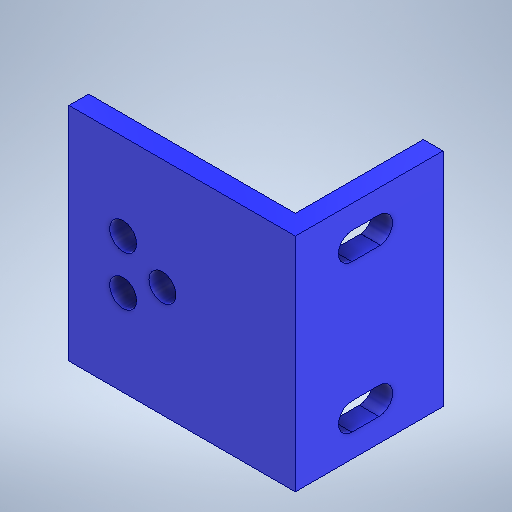
# Autodesk Inventor part: Montagewinkel für Spannelement
Saved by Autodesk Inventor 2025.1 (Build 291241020, 241B)
## iProperties
Created: 2026-05-13
Part Number: Montagewinkel für Spannelement
Material: Generisch
Document SubType Name: Modeling
Designer: pparr
Density: 1 g/cm^3
Appearance: Blau - Wandfarbe - glänzend
Author: pparr
Autodesk Inventor part; units mm, degrees
ref_plane "YZ Plane" through (0, 0, 0) normal (1, 0, 0) x (0, 1, 0)
ref_plane "XZ Plane" through (0, 0, 0) normal (0, 1, 0) x (-1, 0, 0)
ref_plane "XY Plane" through (0, 0, 0) normal (0, 0, 1) x (1, 0, 0)
sketch "Skizze1" plane through (0, 0, 0) normal (1, 0, 0) x (0, 1, 0)
  line L0 (15, 22.5) -> (-15, 22.5)
  line L1 (-15, 22.5) -> (-15, -22.5)
  line L2 (-15, -22.5) -> (15, -22.5)
  line L3 (15, -22.5) -> (15, 22.5)
  line L4 (15, 22.5) -> (-15, -22.5) construction
  line L5 (-15, 22.5) -> (15, -22.5) construction
  point P0 (0, 0)
  dimension "d0" = 30
  dimension "d1" = 45
  constraints: 12 end point, 2 midpoint, 2 parallel, 1 horizontal, 1 perpendicular
  measures "d0" distance of L2.end L1.end
  measures "d1" distance of L1.end L0.end
extrude "Extrusion1" add sketch "Skizze1" along normal blind 4
sketch "Skizze2" plane through (0, 0, 0) normal (-1, 0, 0) x (0, 0, 1)
  line L0 (-22.5, -15) -> (-22.5, 15) projected
  line L1 (-22.5, -11) -> (22.5, -11)
  line L2 (22.5, -11) -> (22.5, -15)
  line L3 (22.5, -15) -> (-22.5, -15)
  line L4 (-22.5, -15) -> (-22.5, -11)
  line L5 (22.5, -15) -> (-22.5, -15) projected
  point P0 (0, 0)
  dimension "d4" = 4
  dimension "d5" = 0
  constraints: 8 end point, 2 parallel, 1 horizontal, 1 perpendicular, 1 point on line
  measures "d4" distance of L1.end L2.end
  measures "d5" distance between parallel lines of L5 L3
extrude "Extrusion2" add sketch "Skizze2" along normal blind 42
sketch "Skizze3" plane through (4, -15, -22.5) normal (0, -1, 0) x (1, 0, 0)
  line L0 (0, 22.5) -> (-45.8958, 22.5)
  line L1 (0, 45) -> (0, 0) projected
  line L2 (-46, 0) -> (-46, 45) projected
  point P0 (-4, 22.5)
  point P1 (-27, 22.5)
  point P2 (-35, 17.5)
  point P3 (-35, 27.5)
  point P4 (-46, 22.5)
  dimension "d15" = 27
  dimension "d17" = 10
  dimension "d18" = 35
  dimension "d19" = 0
  dimension "d21" = 5
  constraints: 2 end point, 2 midpoint, 1 horizontal, 1 point on line
  measures "d15" distance from line of L1 point (-27, 22.5)
  measures "d17" distance of point (-35, 27.5) point (-35, 17.5)
  measures "d18" horizontal distance of point (-35, 17.5) L1.end
  measures "d19" horizontal distance of point (-35, 17.5) point (-35, 27.5)
  measures "d21" vertical distance of point (-35, 17.5) point (-46, 22.5)
hole "Bohrung1" at (-23, -15, 0) at (-31, -15, -5) at (-31, -15, 5) direction (0, 1, 0) diameter 5.5 depth 11.8 tip angle 118
sketch "Skizze5" plane through (0, 0, 0) normal (-1, 0, 0) x (0, 0, 1)
  line L0 (-22.5, -15) -> (22.5, -15) projected
  point P0 (0, 0)
  point P1 (15, -3.5)
  point P2 (-15, -3.5)
  point P3 (15, 2)
  point P4 (-15, 2)
  dimension "d29" = 30
  dimension "d30" = 15
  dimension "d31" = 11.5
  dimension "d32" = 11.5
  dimension "d33" = 15
  dimension "d34" = 30
  dimension "d35" = 5.5
  dimension "d36" = 5.5
  measures "d29" distance of point (-15, -3.5) point (15, -3.5)
  measures "d30" horizontal distance of point (15, -3.5) point (0, 0)
  measures "d31" distance from line of point (15, -3.5) L0
  measures "d32" distance from line of L0 point (-15, -3.5)
  measures "d33" horizontal distance of point (0, 0) point (15, 2)
  measures "d34" distance of point (-15, 2) point (15, 2)
  measures "d35" distance of point (15, 2) point (15, -3.5)
  measures "d36" distance of point (-15, -3.5) point (-15, 2)
hole "Bohrung2" at (0, -3.5, 15) at (0, -3.5, -15) at (0, 2, 15) at (0, 2, -15) direction (1, 0, 0) diameter 5.5 depth 11.8 tip angle 118
sketch "Skizze6" plane through (0, 0, 0) normal (-1, 0, 0) x (0, 0, 1)
  circle A0 centre (15, -3.5) radius 2.75 projected
  line L0 (17.75, -3.5) -> (17.75, 2.2896)
  line L1 (12.25, -3.5) -> (12.25, 2.2896)
  circle A1 centre (-15, -3.5) radius 2.75 projected
  line L2 (-12.25, -3.5) -> (-12.25, 2.2896)
  line L3 (-17.75, -3.5) -> (-17.75, 2)
  circle A2 centre (-15, 2) radius 2.75 projected
  line L4 (17.75, -3.5) -> (12.25, -3.5)
  line L5 (17.75, 2.2896) -> (12.25, 2.2896)
  line L6 (-12.25, -3.5) -> (-17.75, -3.5)
  line L7 (-12.25, 2.2896) -> (-17.7347, 2.2896)
  circle A3 centre (-15, 2) radius 2.75 projected
  point P0 (0, 0)
  point P1 (15, -0.75)
  point P2 (-15, -0.75)
  point P3 (-12.25, 2)
  constraints: 16 end point, 6 point on circle, 4 tangent, 4 vertical, 3 horizontal
extrude "Extrusion3" cut sketch "Skizze6" against normal blind 6 contours A0 L1 L5 L0 | L3 A2 A1 | A1 A2 L2
